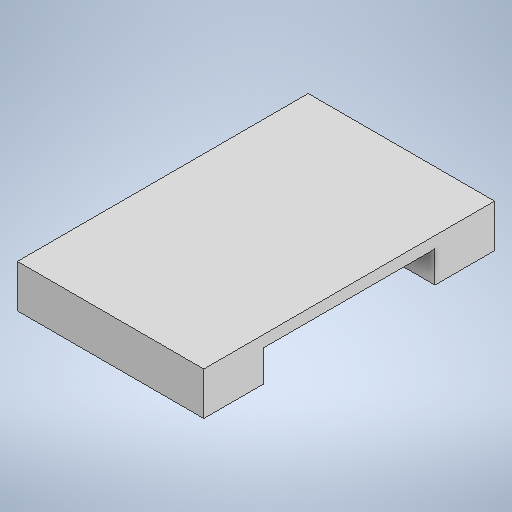
# Autodesk Inventor part: Servo mount top v2
Saved by Autodesk Inventor 2025.2 (Build 292293000, 293)
## iProperties
Created: 2025-01-28
Part Number: Servo mount top v2
Material: Generic
Document SubType Name: Modeling
Designer: Sameer Alhindi
Density: 1 g/cm^3
Appearance: Default
Author: Sameer Alhindi
Autodesk Inventor part; units mm, degrees
ref_plane "YZ Plane" through (0, 0, 0) normal (1, 0, 0) x (0, 1, 0)
ref_plane "XZ Plane" through (0, 0, 0) normal (0, 1, 0) x (-1, 0, 0)
ref_plane "XY Plane" through (0, 0, 0) normal (0, 0, 1) x (1, 0, 0)
sketch "Sketch1" plane through (0, 0, 0) normal (0, 1, 0) x (-1, 0, 0)
  line L0 (0, 0) -> (25, 0)
  line L1 (25, 0) -> (25, -39)
  line L2 (25, -39) -> (0, -39)
  line L3 (0, -39) -> (0, 0)
  line L4 (0, -8) -> (25, -8)
  line L5 (25, -8) -> (25, -31)
  line L6 (25, -31) -> (0, -31)
  line L7 (0, -31) -> (0, -8)
  dimension "d0" = 39
  dimension "d1" = 25
  dimension "d2" = 23
  dimension "d3" = 8
  dimension "d4" = 8
  constraints: 16 end point, 4 parallel, 2 horizontal, 2 perpendicular, 2 point on line
  measures "d0" distance of L2.end L0.start
  measures "d1" distance of L0.start L0.end
  measures "d2" distance between parallel lines of L6 L4
  measures "d3" distance between parallel lines of L0 L4
  measures "d4" distance between parallel lines of L6 L2
extrude "Extrusion1" add sketch "Sketch1" along normal blind 11.5
sketch "Sketch3" plane through (0, 0, 0) normal (1, 0, 0) x (0, 0, -1)
  line L0 (0, 0) -> (0, 11.5) projected
  line L1 (0, 0) -> (39, 0) projected
  line L2 (8, 1.55) -> (31, 1.55)
  line L3 (31, 1.55) -> (31, 9.95)
  line L4 (31, 9.95) -> (8, 9.95)
  line L5 (8, 9.95) -> (8, 1.55)
  line L6 (8, 1.55) -> (31, 9.95) construction
  line L7 (31, 1.55) -> (8, 9.95) construction
  point P0 (0, 5.75)
  point P1 (19.5, 0)
  point P2 (19.5, 5.75)
  dimension "d9" = 23
  dimension "d10" = 8.4
  dimension "d25" = 8
  constraints: 12 end point, 4 midpoint, 2 parallel, 1 horizontal, 1 perpendicular
  measures "d9" distance of L4.end L3.end
  measures "d10" distance of L2.end L3.end
  measures "d25" distance from line of point (0, 5.75) L5
extrude "Extrusion2" cut sketch "Sketch3" against normal through all
sketch "Sketch4" plane through (0, 0, 0) normal (1, 0, 0) x (0, 0, -1)
  line L0 (0, 0) -> (0, 11.5) projected
  line L1 (0, 5.75) -> (39, 5.75)
  line L2 (39, 0) -> (39, 11.5) projected
  constraints: 2 end point, 2 midpoint
split body "Split1" sketch "Sketch4" result one side removed curves L1 removed pieces at (-8.3333, 0.5, -13)
body "Solid1"
